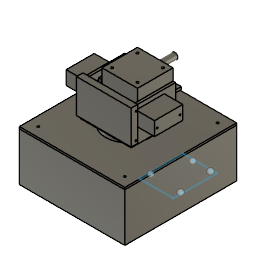
carro_armato_assieme_completo_modificabile_v3_batteria_integrata_canale_cavi (Autodesk Fusion 360 design; units mm, degrees)
part number: 2026-07-14-00-47-27-099
part number: 2026-07-14-00-47-27-347
part number: 2026-07-14-00-47-27-486
part number: 2026-07-14-00-47-29-459
part number: 2026-07-14-00-47-30-510
part number: 2026-07-14-00-47-30-620
part number: 2026-07-14-00-47-31-160
part number: 2026-07-14-00-47-33-248
part number: 2026-07-14-00-47-33-746
part number: 2026-07-14-00-47-35-683
part number: 2026-07-14-00-47-43-018
part number: 2026-07-14-00-47-43-807
part number: 2026-07-14-00-47-44-634
part number: 2026-07-14-00-47-46-224
part number: 2026-07-14-00-47-47-931
part number: 2026-07-14-00-47-54-379
part number: 2026-07-14-00-47-59-132
part number: 2026-07-14-00-48-06-266
part number: 2026-07-14-00-48-10-461
part number: 2026-07-14-00-48-14-735
Autodesk Fusion 360 part; units mm, degrees
(part 1 of 2)
sketch "Schizzo1" plane through (0, 0, 0) normal (0, 0, 1) x (1, 0, 0) in component "01_Piano_inferiore_colonnine_M3_supporto_batteria_integrato"
  line L0 (-80, -85) -> (80, -85)
  line L1 (80, -85) -> (80, 85)
  line L2 (80, 85) -> (-80, 85)
  line L3 (-80, 85) -> (-80, -85)
extrude "Estrusione_Piano_inferiore" add sketch "Schizzo1" along normal blind 3 makes body 1 in component "01_Piano_inferiore_colonnine_M3_supporto_batteria_integrato"
ref_plane "Piano di lavoro1" through (0, 0, 43) normal (0, 0, 1) x (1, 0, 0) in component "02_Piano_superiore"
sketch "Schizzo1 (2)" plane through (0, 0, 43) normal (0, 0, 1) x (1, 0, 0) in component "02_Piano_superiore"
  line L0 (-80, -85) -> (80, -85)
  line L1 (80, -85) -> (80, 85)
  line L2 (80, 85) -> (-80, 85)
  line L3 (-80, 85) -> (-80, -85)
extrude "Estrusione_Piano_superiore" add sketch "Schizzo1 (2)" along normal blind 3 separate body makes body 2 in component "02_Piano_superiore"
ref_plane "Piano di lavoro1" through (0, 0, 3) normal (0, 0, 1) x (1, 0, 0) in component "01_Piano_inferiore_colonnine_M3_supporto_batteria_integrato"
ref_plane "Piano di lavoro2" through (0, 0, 40.4) normal (0, 0, 1) x (1, 0, 0) in component "01_Piano_inferiore_colonnine_M3_supporto_batteria_integrato"
sketch "Schizzo2" plane through (0, 0, 0) normal (0, 0, 1) x (1, 0, 0) in component "01_Piano_inferiore_colonnine_M3_supporto_batteria_integrato"
  line L0 (-5, -77.5) -> (5, -77.5)
  line L1 (5, -77.5) -> (5, -72.5)
  line L2 (5, -72.5) -> (-5, -72.5)
  line L3 (-5, -72.5) -> (-5, -77.5)
extrude "Asola_fascetta_01" cut sketch "Schizzo2" along normal blind 3 bodies 1 in component "01_Piano_inferiore_colonnine_M3_supporto_batteria_integrato"
sketch "Schizzo3" plane through (0, 0, 0) normal (0, 0, 1) x (1, 0, 0) in component "01_Piano_inferiore_colonnine_M3_supporto_batteria_integrato"
  line L0 (-5, -62.5) -> (5, -62.5)
  line L1 (5, -62.5) -> (5, -57.5)
  line L2 (5, -57.5) -> (-5, -57.5)
  line L3 (-5, -57.5) -> (-5, -62.5)
extrude "Asola_fascetta_02" cut sketch "Schizzo3" along normal blind 3 bodies 1 in component "01_Piano_inferiore_colonnine_M3_supporto_batteria_integrato"
sketch "Schizzo4" plane through (0, 0, 0) normal (0, 0, 1) x (1, 0, 0) in component "01_Piano_inferiore_colonnine_M3_supporto_batteria_integrato"
  line L0 (-5, -12.5) -> (5, -12.5)
  line L1 (5, -12.5) -> (5, -7.5)
  line L2 (5, -7.5) -> (-5, -7.5)
  line L3 (-5, -7.5) -> (-5, -12.5)
extrude "Asola_fascetta_03" cut sketch "Schizzo4" along normal blind 3 bodies 1 in component "01_Piano_inferiore_colonnine_M3_supporto_batteria_integrato"
sketch "Schizzo5" plane through (0, 0, 0) normal (0, 0, 1) x (1, 0, 0) in component "01_Piano_inferiore_colonnine_M3_supporto_batteria_integrato"
  line L0 (-5, 2.5) -> (5, 2.5)
  line L1 (5, 2.5) -> (5, 7.5)
  line L2 (5, 7.5) -> (-5, 7.5)
  line L3 (-5, 7.5) -> (-5, 2.5)
extrude "Asola_fascetta_04" cut sketch "Schizzo5" along normal blind 3 bodies 1 in component "01_Piano_inferiore_colonnine_M3_supporto_batteria_integrato"
sketch "Schizzo2 (2)" plane through (0, 0, 43) normal (0, 0, 1) x (1, 0, 0) in component "02_Piano_superiore"
  circle A0 centre (-68, -73) radius 1.6
extrude "Foro_M3_superiore_01" cut sketch "Schizzo2 (2)" along normal blind 3 bodies 2 in component "02_Piano_superiore"
sketch "Schizzo6" plane through (0, 0, 3) normal (0, 0, 1) x (1, 0, 0) in component "01_Piano_inferiore_colonnine_M3_supporto_batteria_integrato"
  circle A0 centre (-68, -73) radius 5
extrude "Estrusione_Colonnina_M3_01" add sketch "Schizzo6" along normal blind 40 bodies 1 in component "01_Piano_inferiore_colonnine_M3_supporto_batteria_integrato"
sketch "Schizzo7" plane through (0, 0, 0) normal (0, 0, 1) x (1, 0, 0) in component "01_Piano_inferiore_colonnine_M3_supporto_batteria_integrato"
  circle A0 centre (-68, -73) radius 1.6
extrude "Foro_passante_M3_colonnina_01" cut sketch "Schizzo7" along normal blind 43 bodies 1 in component "01_Piano_inferiore_colonnine_M3_supporto_batteria_integrato"
sketch "Schizzo8" plane through (0, 0, 40.4) normal (0, 0, 1) x (1, 0, 0) in component "01_Piano_inferiore_colonnine_M3_supporto_batteria_integrato"
  line L0 (-65.1, -71.3257) -> (-68, -69.6514)
  line L1 (-68, -69.6514) -> (-70.9, -71.3257)
  line L2 (-70.9, -71.3257) -> (-70.9, -74.6743)
  line L3 (-70.9, -74.6743) -> (-68, -76.3486)
  line L4 (-68, -76.3486) -> (-65.1, -74.6743)
  line L5 (-65.1, -74.6743) -> (-65.1, -71.3257)
extrude "Sede_dado_M3_01" cut sketch "Schizzo8" along normal blind 2.6 bodies 1 in component "01_Piano_inferiore_colonnine_M3_supporto_batteria_integrato"
sketch "Schizzo3 (2)" plane through (0, 0, 43) normal (0, 0, 1) x (1, 0, 0) in component "02_Piano_superiore"
  circle A0 centre (68, -73) radius 1.6
extrude "Foro_M3_superiore_02" cut sketch "Schizzo3 (2)" along normal blind 3 bodies 2 in component "02_Piano_superiore"
sketch "Schizzo9" plane through (0, 0, 3) normal (0, 0, 1) x (1, 0, 0) in component "01_Piano_inferiore_colonnine_M3_supporto_batteria_integrato"
  circle A0 centre (68, -73) radius 5
extrude "Estrusione_Colonnina_M3_02" add sketch "Schizzo9" along normal blind 40 bodies 1 in component "01_Piano_inferiore_colonnine_M3_supporto_batteria_integrato"
sketch "Schizzo10" plane through (0, 0, 0) normal (0, 0, 1) x (1, 0, 0) in component "01_Piano_inferiore_colonnine_M3_supporto_batteria_integrato"
  circle A0 centre (68, -73) radius 1.6
extrude "Foro_passante_M3_colonnina_02" cut sketch "Schizzo10" along normal blind 43 bodies 1 in component "01_Piano_inferiore_colonnine_M3_supporto_batteria_integrato"
sketch "Schizzo11" plane through (0, 0, 40.4) normal (0, 0, 1) x (1, 0, 0) in component "01_Piano_inferiore_colonnine_M3_supporto_batteria_integrato"
  line L0 (70.9, -71.3257) -> (68, -69.6514)
  line L1 (68, -69.6514) -> (65.1, -71.3257)
  line L2 (65.1, -71.3257) -> (65.1, -74.6743)
  line L3 (65.1, -74.6743) -> (68, -76.3486)
  line L4 (68, -76.3486) -> (70.9, -74.6743)
  line L5 (70.9, -74.6743) -> (70.9, -71.3257)
extrude "Sede_dado_M3_02" cut sketch "Schizzo11" along normal blind 2.6 bodies 1 in component "01_Piano_inferiore_colonnine_M3_supporto_batteria_integrato"
sketch "Schizzo4 (2)" plane through (0, 0, 43) normal (0, 0, 1) x (1, 0, 0) in component "02_Piano_superiore"
  circle A0 centre (68, 73) radius 1.6
extrude "Foro_M3_superiore_03" cut sketch "Schizzo4 (2)" along normal blind 3 bodies 2 in component "02_Piano_superiore"
sketch "Schizzo12" plane through (0, 0, 3) normal (0, 0, 1) x (1, 0, 0) in component "01_Piano_inferiore_colonnine_M3_supporto_batteria_integrato"
  circle A0 centre (68, 73) radius 5
extrude "Estrusione_Colonnina_M3_03" add sketch "Schizzo12" along normal blind 40 bodies 1 in component "01_Piano_inferiore_colonnine_M3_supporto_batteria_integrato"
sketch "Schizzo13" plane through (0, 0, 0) normal (0, 0, 1) x (1, 0, 0) in component "01_Piano_inferiore_colonnine_M3_supporto_batteria_integrato"
  circle A0 centre (68, 73) radius 1.6
extrude "Foro_passante_M3_colonnina_03" cut sketch "Schizzo13" along normal blind 43 bodies 1 in component "01_Piano_inferiore_colonnine_M3_supporto_batteria_integrato"
sketch "Schizzo14" plane through (0, 0, 40.4) normal (0, 0, 1) x (1, 0, 0) in component "01_Piano_inferiore_colonnine_M3_supporto_batteria_integrato"
  line L0 (70.9, 74.6743) -> (68, 76.3486)
  line L1 (68, 76.3486) -> (65.1, 74.6743)
  line L2 (65.1, 74.6743) -> (65.1, 71.3257)
  line L3 (65.1, 71.3257) -> (68, 69.6514)
  line L4 (68, 69.6514) -> (70.9, 71.3257)
  line L5 (70.9, 71.3257) -> (70.9, 74.6743)
extrude "Sede_dado_M3_03" cut sketch "Schizzo14" along normal blind 2.6 bodies 1 in component "01_Piano_inferiore_colonnine_M3_supporto_batteria_integrato"
sketch "Schizzo5 (2)" plane through (0, 0, 43) normal (0, 0, 1) x (1, 0, 0) in component "02_Piano_superiore"
  circle A0 centre (-68, 73) radius 1.6
extrude "Foro_M3_superiore_04" cut sketch "Schizzo5 (2)" along normal blind 3 bodies 2 in component "02_Piano_superiore"
sketch "Schizzo15" plane through (0, 0, 3) normal (0, 0, 1) x (1, 0, 0) in component "01_Piano_inferiore_colonnine_M3_supporto_batteria_integrato"
  circle A0 centre (-68, 73) radius 5
extrude "Estrusione_Colonnina_M3_04" add sketch "Schizzo15" along normal blind 40 bodies 1 in component "01_Piano_inferiore_colonnine_M3_supporto_batteria_integrato"
sketch "Schizzo16" plane through (0, 0, 0) normal (0, 0, 1) x (1, 0, 0) in component "01_Piano_inferiore_colonnine_M3_supporto_batteria_integrato"
  circle A0 centre (-68, 73) radius 1.6
extrude "Foro_passante_M3_colonnina_04" cut sketch "Schizzo16" along normal blind 43 bodies 1 in component "01_Piano_inferiore_colonnine_M3_supporto_batteria_integrato"
sketch "Schizzo17" plane through (0, 0, 40.4) normal (0, 0, 1) x (1, 0, 0) in component "01_Piano_inferiore_colonnine_M3_supporto_batteria_integrato"
  line L0 (-65.1, 74.6743) -> (-68, 76.3486)
  line L1 (-68, 76.3486) -> (-70.9, 74.6743)
  line L2 (-70.9, 74.6743) -> (-70.9, 71.3257)
  line L3 (-70.9, 71.3257) -> (-68, 69.6514)
  line L4 (-68, 69.6514) -> (-65.1, 71.3257)
  line L5 (-65.1, 71.3257) -> (-65.1, 74.6743)
extrude "Sede_dado_M3_04" cut sketch "Schizzo17" along normal blind 2.6 bodies 1 in component "01_Piano_inferiore_colonnine_M3_supporto_batteria_integrato"
sketch "Schizzo6 (2)" plane through (0, 0, 43) normal (0, 0, 1) x (1, 0, 0) in component "02_Piano_superiore"
  line L0 (20.83, 33.21) -> (45.83, 33.21)
  line L1 (45.83, 33.21) -> (45.83, 58.21)
  line L2 (45.83, 58.21) -> (20.83, 58.21)
  line L3 (20.83, 58.21) -> (20.83, 33.21)
extrude "Apertura_Arduino_25x25_D2_D7_S1_S8" cut sketch "Schizzo6 (2)" along normal blind 3 bodies 2 in component "02_Piano_superiore"
sketch "Schizzo7 (2)" plane through (0, 0, 43) normal (0, 0, 1) x (1, 0, 0) in component "02_Piano_superiore"
  line L0 (-69, -45) -> (-36, -45)
  line L1 (-36, -45) -> (-36, 15)
  line L2 (-36, 15) -> (-69, 15)
  line L3 (-69, 15) -> (-69, -45)
extrude "Apertura_pacco_batteria_PCB_cannone_60x33" cut sketch "Schizzo7 (2)" along normal blind 3 bodies 2 in component "02_Piano_superiore"
sketch "Schizzo8 (2)" plane through (0, 0, 43) normal (0, 0, 1) x (1, 0, 0) in component "02_Piano_superiore"
  circle A0 centre (0, -79.5) radius 1.35
extrude "Foro_M2_5_guscio_inferiore_01_south" cut sketch "Schizzo8 (2)" along normal blind 3 bodies 2 in component "02_Piano_superiore"
sketch "Schizzo9 (2)" plane through (0, 0, 43) normal (0, 0, 1) x (1, 0, 0) in component "02_Piano_superiore"
  circle A0 centre (0, 79.5) radius 1.35
extrude "Foro_M2_5_guscio_inferiore_02_north" cut sketch "Schizzo9 (2)" along normal blind 3 bodies 2 in component "02_Piano_superiore"
sketch "Schizzo10 (2)" plane through (0, 0, 43) normal (0, 0, 1) x (1, 0, 0) in component "02_Piano_superiore"
  circle A0 centre (74.5, 45) radius 1.35
extrude "Foro_M2_5_guscio_inferiore_03_east" cut sketch "Schizzo10 (2)" along normal blind 3 bodies 2 in component "02_Piano_superiore"
sketch "Schizzo11 (2)" plane through (0, 0, 43) normal (0, 0, 1) x (1, 0, 0) in component "02_Piano_superiore"
  circle A0 centre (-74.5, 45) radius 1.35
extrude "Foro_M2_5_guscio_inferiore_04_west" cut sketch "Schizzo11 (2)" along normal blind 3 bodies 2 in component "02_Piano_superiore"
ref_plane "Piano di lavoro3" through (0, 0, 3) normal (0, 0, 1) x (1, 0, 0) in component "01_Piano_inferiore_colonnine_M3_supporto_batteria_integrato"
sketch "Schizzo18" plane through (0, 0, 3) normal (0, 0, 1) x (1, 0, 0) in component "01_Piano_inferiore_colonnine_M3_supporto_batteria_integrato"
  line L0 (-75, -65) -> (-72.5, -65)
  line L1 (-72.5, -65) -> (-72.5, 35)
  line L2 (-72.5, 35) -> (-75, 35)
  line L3 (-75, 35) -> (-75, -65)
extrude "Estrusione_Parete_lunga_Ovest" add sketch "Schizzo18" along normal blind 17 bodies 1 in component "01_Piano_inferiore_colonnine_M3_supporto_batteria_integrato"
sketch "Schizzo19" plane through (0, 0, 3) normal (0, 0, 1) x (1, 0, 0) in component "01_Piano_inferiore_colonnine_M3_supporto_batteria_integrato"
  line L0 (-32.5, -65) -> (-30, -65)
  line L1 (-30, -65) -> (-30, 35)
  line L2 (-30, 35) -> (-32.5, 35)
  line L3 (-32.5, 35) -> (-32.5, -65)
extrude "Estrusione_Parete_lunga_Est" add sketch "Schizzo19" along normal blind 17 bodies 1 in component "01_Piano_inferiore_colonnine_M3_supporto_batteria_integrato"
sketch "Schizzo20" plane through (0, 0, 3) normal (0, 0, 1) x (1, 0, 0) in component "01_Piano_inferiore_colonnine_M3_supporto_batteria_integrato"
  line L0 (-75, -65) -> (-30, -65)
  line L1 (-30, -65) -> (-30, -60)
  line L2 (-30, -60) -> (-75, -60)
  line L3 (-75, -60) -> (-75, -65)
extrude "Estrusione_Parete_corta_chiusa" add sketch "Schizzo20" along normal blind 17 bodies 1 in component "01_Piano_inferiore_colonnine_M3_supporto_batteria_integrato"
sketch "Schizzo21" plane through (0, 0, 3) normal (0, 0, 1) x (1, 0, 0) in component "01_Piano_inferiore_colonnine_M3_supporto_batteria_integrato"
  line L0 (-32.6, -60) -> (-29.9, -60)
  line L1 (-29.9, -60) -> (-29.9, -50)
  line L2 (-29.9, -50) -> (-32.6, -50)
  line L3 (-32.6, -50) -> (-32.6, -60)
extrude "Apertura_cavi_parete_lunga_Est" cut sketch "Schizzo21" along normal blind 17 bodies 1 in component "01_Piano_inferiore_colonnine_M3_supporto_batteria_integrato"
sketch "Schizzo1 (3)" plane through (0, 0, 0) normal (0, 0, 1) x (1, 0, 0) in component "03_Guscio_laterale_continuo_carro"
  line L0 (-83, -88) -> (-80.5, -88)
  line L1 (-80.5, -88) -> (-80.5, 88)
  line L2 (-80.5, 88) -> (-83, 88)
  line L3 (-83, 88) -> (-83, -88)
extrude "Estrusione_Parete_guscio_Ovest" add sketch "Schizzo1 (3)" along normal blind 76 separate body makes body 3 in component "03_Guscio_laterale_continuo_carro"
sketch "Schizzo2 (3)" plane through (0, 0, 0) normal (0, 0, 1) x (1, 0, 0) in component "03_Guscio_laterale_continuo_carro"
  line L0 (-83, -88) -> (83, -88)
  line L1 (83, -88) -> (83, -85.5)
  line L2 (83, -85.5) -> (-83, -85.5)
  line L3 (-83, -85.5) -> (-83, -88)
extrude "Estrusione_Parete_guscio_Sud" add sketch "Schizzo2 (3)" along normal blind 76 bodies 3 in component "03_Guscio_laterale_continuo_carro"
sketch "Schizzo3 (3)" plane through (0, 0, 0) normal (0, 0, 1) x (1, 0, 0) in component "03_Guscio_laterale_continuo_carro"
  line L0 (80.5, -88) -> (83, -88)
  line L1 (83, -88) -> (83, 88)
  line L2 (83, 88) -> (80.5, 88)
  line L3 (80.5, 88) -> (80.5, -88)
extrude "Estrusione_Parete_guscio_Est" add sketch "Schizzo3 (3)" along normal blind 76 bodies 3 in component "03_Guscio_laterale_continuo_carro"
sketch "Schizzo4 (3)" plane through (0, 0, 0) normal (0, 0, 1) x (1, 0, 0) in component "03_Guscio_laterale_continuo_carro"
  line L0 (-83, 85.5) -> (83, 85.5)
  line L1 (83, 85.5) -> (83, 88)
  line L2 (83, 88) -> (-83, 88)
  line L3 (-83, 88) -> (-83, 85.5)
extrude "Estrusione_Parete_guscio_Nord" add sketch "Schizzo4 (3)" along normal blind 76 bodies 3 in component "03_Guscio_laterale_continuo_carro"
ref_plane "Piano di lavoro1" through (0, 0, 38) normal (0, 0, 1) x (1, 0, 0) in component "03_Guscio_laterale_continuo_carro"
sketch "Schizzo5 (3)" plane through (0, 0, 38) normal (0, 0, 1) x (1, 0, 0) in component "03_Guscio_laterale_continuo_carro"
  line L0 (-7, -86) -> (7, -86)
  line L1 (7, -86) -> (7, -73)
  line L2 (7, -73) -> (-7, -73)
  line L3 (-7, -73) -> (-7, -86)
extrude "Estrusione_Linguetta_M2_5_01_south" add sketch "Schizzo5 (3)" along normal blind 5 bodies 3 in component "03_Guscio_laterale_continuo_carro"
sketch "Schizzo6 (3)" plane through (0, 0, 38) normal (0, 0, 1) x (1, 0, 0) in component "03_Guscio_laterale_continuo_carro"
  circle A0 centre (0, -79.5) radius 1.1
extrude "Preforo_M2_5_guscio_01_south" cut sketch "Schizzo6 (3)" along normal blind 5 bodies 3 in component "03_Guscio_laterale_continuo_carro"
sketch "Schizzo7 (3)" plane through (0, 0, 38) normal (0, 0, 1) x (1, 0, 0) in component "03_Guscio_laterale_continuo_carro"
  line L0 (-7, 73) -> (7, 73)
  line L1 (7, 73) -> (7, 86)
  line L2 (7, 86) -> (-7, 86)
  line L3 (-7, 86) -> (-7, 73)
extrude "Estrusione_Linguetta_M2_5_02_north" add sketch "Schizzo7 (3)" along normal blind 5 bodies 3 in component "03_Guscio_laterale_continuo_carro"
sketch "Schizzo8 (3)" plane through (0, 0, 38) normal (0, 0, 1) x (1, 0, 0) in component "03_Guscio_laterale_continuo_carro"
  circle A0 centre (0, 79.5) radius 1.1
extrude "Preforo_M2_5_guscio_02_north" cut sketch "Schizzo8 (3)" along normal blind 5 bodies 3 in component "03_Guscio_laterale_continuo_carro"
sketch "Schizzo9 (3)" plane through (0, 0, 38) normal (0, 0, 1) x (1, 0, 0) in component "03_Guscio_laterale_continuo_carro"
  line L0 (68, 38) -> (81, 38)
  line L1 (81, 38) -> (81, 52)
  line L2 (81, 52) -> (68, 52)
  line L3 (68, 52) -> (68, 38)
extrude "Estrusione_Linguetta_M2_5_03_east" add sketch "Schizzo9 (3)" along normal blind 5 bodies 3 in component "03_Guscio_laterale_continuo_carro"
sketch "Schizzo10 (3)" plane through (0, 0, 38) normal (0, 0, 1) x (1, 0, 0) in component "03_Guscio_laterale_continuo_carro"
  circle A0 centre (74.5, 45) radius 1.1
extrude "Preforo_M2_5_guscio_03_east" cut sketch "Schizzo10 (3)" along normal blind 5 bodies 3 in component "03_Guscio_laterale_continuo_carro"
sketch "Schizzo11 (3)" plane through (0, 0, 38) normal (0, 0, 1) x (1, 0, 0) in component "03_Guscio_laterale_continuo_carro"
  line L0 (-81, 38) -> (-68, 38)
  line L1 (-68, 38) -> (-68, 52)
  line L2 (-68, 52) -> (-81, 52)
  line L3 (-81, 52) -> (-81, 38)
extrude "Estrusione_Linguetta_M2_5_04_west" add sketch "Schizzo11 (3)" along normal blind 5 bodies 3 in component "03_Guscio_laterale_continuo_carro"
sketch "Schizzo12 (2)" plane through (0, 0, 38) normal (0, 0, 1) x (1, 0, 0) in component "03_Guscio_laterale_continuo_carro"
  circle A0 centre (-74.5, 45) radius 1.1
extrude "Preforo_M2_5_guscio_04_west" cut sketch "Schizzo12 (2)" along normal blind 5 bodies 3 in component "03_Guscio_laterale_continuo_carro"
sketch "Schizzo1 (4)" plane through (0, 0, 0) normal (0, 0, 1) x (1, 0, 0) in component "05_Arduino_UNO_R4_WiFi_RIFERIMENTO_XY_quota_Z_da_definire"
  line L0 (-26.67, -34.29) -> (26.67, -34.29)
  line L1 (26.67, -34.29) -> (26.67, 34.29)
  line L2 (26.67, 34.29) -> (-26.67, 34.29)
  line L3 (-26.67, 34.29) -> (-26.67, -34.29)
  circle A0 centre (24.13, -20.32) radius 1.6
  circle A1 centre (-24.13, -19.05) radius 1.6
  circle A2 centre (19.05, 31.75) radius 1.6
  circle A3 centre (-8.89, 31.75) radius 1.6
ref_plane "Piano di lavoro1" through (0, 0, 30) normal (0, 0, 1) x (1, 0, 0) in component "01_Tetto_elettronica_removibile"
sketch "Schizzo1 (5)" plane through (0, 0, 30) normal (0, 0, 1) x (1, 0, 0) in component "01_Tetto_elettronica_removibile"
  line L0 (-83, -88) -> (83, -88)
  line L1 (83, -88) -> (83, 88)
  line L2 (83, 88) -> (-83, 88)
  line L3 (-83, 88) -> (-83, -88)
extrude "Estrusione_Tetto_coperchio" add sketch "Schizzo1 (5)" along normal blind 3 separate body makes body 4 in component "01_Tetto_elettronica_removibile"
sketch "Schizzo2 (4)" plane through (0, 0, 0) normal (0, 0, 1) x (1, 0, 0) in component "01_Tetto_elettronica_removibile"
  circle A0 centre (-68, -73) radius 5
extrude "Estrusione_Boss_verticale_M3_coperchio_01" add sketch "Schizzo2 (4)" along normal blind 33 bodies 4 in component "01_Tetto_elettronica_removibile"
sketch "Schizzo3 (4)" plane through (0, 0, 0) normal (0, 0, 1) x (1, 0, 0) in component "01_Tetto_elettronica_removibile"
  circle A0 centre (-68, -73) radius 1.6
extrude "Foro_M3_accessibile_dal_tetto_01" cut sketch "Schizzo3 (4)" along normal blind 33 bodies 4 in component "01_Tetto_elettronica_removibile"
sketch "Schizzo4 (4)" plane through (0, 0, 0) normal (0, 0, 1) x (1, 0, 0) in component "01_Tetto_elettronica_removibile"
  circle A0 centre (68, -73) radius 5
extrude "Estrusione_Boss_verticale_M3_coperchio_02" add sketch "Schizzo4 (4)" along normal blind 33 bodies 4 in component "01_Tetto_elettronica_removibile"
sketch "Schizzo5 (4)" plane through (0, 0, 0) normal (0, 0, 1) x (1, 0, 0) in component "01_Tetto_elettronica_removibile"
  circle A0 centre (68, -73) radius 1.6
extrude "Foro_M3_accessibile_dal_tetto_02" cut sketch "Schizzo5 (4)" along normal blind 33 bodies 4 in component "01_Tetto_elettronica_removibile"
sketch "Schizzo6 (4)" plane through (0, 0, 0) normal (0, 0, 1) x (1, 0, 0) in component "01_Tetto_elettronica_removibile"
  circle A0 centre (-68, 73) radius 5
extrude "Estrusione_Boss_verticale_M3_coperchio_03" add sketch "Schizzo6 (4)" along normal blind 33 bodies 4 in component "01_Tetto_elettronica_removibile"
sketch "Schizzo7 (4)" plane through (0, 0, 0) normal (0, 0, 1) x (1, 0, 0) in component "01_Tetto_elettronica_removibile"
  circle A0 centre (-68, 73) radius 1.6
extrude "Foro_M3_accessibile_dal_tetto_03" cut sketch "Schizzo7 (4)" along normal blind 33 bodies 4 in component "01_Tetto_elettronica_removibile"
sketch "Schizzo8 (4)" plane through (0, 0, 0) normal (0, 0, 1) x (1, 0, 0) in component "01_Tetto_elettronica_removibile"
  circle A0 centre (68, 73) radius 5
extrude "Estrusione_Boss_verticale_M3_coperchio_04" add sketch "Schizzo8 (4)" along normal blind 33 bodies 4 in component "01_Tetto_elettronica_removibile"
sketch "Schizzo9 (4)" plane through (0, 0, 0) normal (0, 0, 1) x (1, 0, 0) in component "01_Tetto_elettronica_removibile"
  circle A0 centre (68, 73) radius 1.6
extrude "Foro_M3_accessibile_dal_tetto_04" cut sketch "Schizzo9 (4)" along normal blind 33 bodies 4 in component "01_Tetto_elettronica_removibile"
ref_plane "Piano di lavoro2" through (0, 0, 30) normal (0, 0, 1) x (1, 0, 0) in component "01_Tetto_elettronica_removibile"
sketch "Schizzo10 (4)" plane through (0, 0, 30) normal (0, 0, 1) x (1, 0, 0) in component "01_Tetto_elettronica_removibile"
  circle A0 centre (0, 0) radius 4
extrude "Passaggio_albero_stepper" cut sketch "Schizzo10 (4)" along normal blind 3 bodies 4 in component "01_Tetto_elettronica_removibile"
sketch "Schizzo11 (4)" plane through (0, 0, 30) normal (0, 0, 1) x (1, 0, 0) in component "01_Tetto_elettronica_removibile"
  circle A0 centre (-17.5, 0) radius 2.1
extrude "Foro_stepper_Ovest" cut sketch "Schizzo11 (4)" along normal blind 3 bodies 4 in component "01_Tetto_elettronica_removibile"
sketch "Schizzo12 (3)" plane through (0, 0, 30) normal (0, 0, 1) x (1, 0, 0) in component "01_Tetto_elettronica_removibile"
  circle A0 centre (17.5, 0) radius 2.1
extrude "Foro_stepper_Est" cut sketch "Schizzo12 (3)" along normal blind 3 bodies 4 in component "01_Tetto_elettronica_removibile"
ref_plane "Piano di lavoro3" through (0, 0, 22.8) normal (0, 0, 1) x (1, 0, 0) in component "01_Tetto_elettronica_removibile"
sketch "Schizzo13 (2)" plane through (0, 0, 22.8) normal (0, 0, 1) x (1, 0, 0) in component "01_Tetto_elettronica_removibile"
  circle A0 centre (0, 0) radius 24
  circle A1 centre (0, 0) radius 22.5
extrude "Estrusione_Parete_interna_liscia_canale_cavi" add sketch "Schizzo13 (2)" along normal blind 7.4 bodies 4 in component "01_Tetto_elettronica_removibile"
sketch "Schizzo14 (2)" plane through (0, 0, 22.8) normal (0, 0, 1) x (1, 0, 0) in component "01_Tetto_elettronica_removibile"
  circle A0 centre (0, 0) radius 33.5
  circle A1 centre (0, 0) radius 32
extrude "Estrusione_Parete_esterna_liscia_canale_cavi" add sketch "Schizzo14 (2)" along normal blind 7.4 bodies 4 in component "01_Tetto_elettronica_removibile"
ref_plane "Piano di lavoro4" through (0, 0, 20) normal (0, 0, 1) x (1, 0, 0) in component "01_Tetto_elettronica_removibile"
sketch "Schizzo15 (2)" plane through (0, 0, 20) normal (0, 0, 1) x (1, 0, 0) in component "01_Tetto_elettronica_removibile"
  circle A0 centre (0, 0) radius 40
  circle A1 centre (0, 0) radius 19
extrude "Estrusione_Fondo_anulare_continuo_canale_cavi" add sketch "Schizzo15 (2)" along normal blind 3 bodies 4 in component "01_Tetto_elettronica_removibile"
sketch "Schizzo16 (2)" plane through (0, 0, 20) normal (0, 0, 1) x (1, 0, 0) in component "01_Tetto_elettronica_removibile"
  line L0 (19.0919, 14.8492) -> (24.7487, 20.5061)
  line L1 (24.7487, 20.5061) -> (20.5061, 24.7487)
  line L2 (20.5061, 24.7487) -> (14.8492, 19.0919)
  line L3 (14.8492, 19.0919) -> (19.0919, 14.8492)
extrude "Uscita_fissa_8x6_canale_cavi_verso_vano_elettronica" cut sketch "Schizzo16 (2)" along normal blind 3 bodies 4 in component "01_Tetto_elettronica_removibile"
sketch "Schizzo17 (2)" plane through (0, 0, 30) normal (0, 0, 1) x (1, 0, 0) in component "01_Tetto_elettronica_removibile"
  circle A0 centre (0, 0) radius 32
  circle A1 centre (0, 0) radius 24
extrude "Guida_anulare_cavi_azimut_meno180_piu180" cut sketch "Schizzo17 (2)" along normal blind 3 bodies 4 in component "01_Tetto_elettronica_removibile"
ref_plane "Piano di lavoro1" through (0, 0, 10) normal (0, 0, 1) x (1, 0, 0) in component "02_Stepper_28BYJ48_riferimento"
sketch "Schizzo1 (6)" plane through (0, 0, 10) normal (0, 0, 1) x (1, 0, 0) in component "02_Stepper_28BYJ48_riferimento"
  circle A0 centre (0, 0) radius 14
extrude "Estrusione_Corpo_stepper" add sketch "Schizzo1 (6)" along normal blind 20 separate body makes body 5 in component "02_Stepper_28BYJ48_riferimento"
ref_plane "Piano di lavoro2" through (0, 0, 27) normal (0, 0, 1) x (1, 0, 0) in component "02_Stepper_28BYJ48_riferimento"
sketch "Schizzo2 (5)" plane through (0, 0, 27) normal (0, 0, 1) x (1, 0, 0) in component "02_Stepper_28BYJ48_riferimento"
  line L0 (-20.75, -4) -> (20.75, -4)
  line L1 (20.75, -4) -> (20.75, 4)
  line L2 (20.75, 4) -> (-20.75, 4)
  line L3 (-20.75, 4) -> (-20.75, -4)
extrude "Estrusione_Alette_fissaggio_stepper" add sketch "Schizzo2 (5)" along normal blind 3 bodies 5 in component "02_Stepper_28BYJ48_riferimento"
ref_plane "Piano di lavoro3" through (0, 0, 30) normal (0, 0, 1) x (1, 0, 0) in component "02_Stepper_28BYJ48_riferimento"
sketch "Schizzo3 (5)" plane through (0, 0, 30) normal (0, 0, 1) x (1, 0, 0) in component "02_Stepper_28BYJ48_riferimento"
  circle A0 centre (0, 0) radius 2.5
extrude "Estrusione_Albero_stepper" add sketch "Schizzo3 (5)" along normal blind 9 bodies 5 in component "02_Stepper_28BYJ48_riferimento"
ref_plane "Piano di lavoro1" through (0, 0, 33) normal (0, 0, 1) x (1, 0, 0) in component "03_Adattatore_rotante_stepper"
sketch "Schizzo1 (7)" plane through (0, 0, 33) normal (0, 0, 1) x (1, 0, 0) in component "03_Adattatore_rotante_stepper"
  circle A0 centre (0, 0) radius 35
extrude "Estrusione_Piastra_adattatore_rotante" add sketch "Schizzo1 (7)" along normal blind 6 separate body makes body 6 in component "03_Adattatore_rotante_stepper"
sketch "Schizzo2 (6)" plane through (0, 0, 33) normal (0, 0, 1) x (1, 0, 0) in component "03_Adattatore_rotante_stepper"
  circle A0 centre (0, 0) radius 2.65
extrude "Sede_albero_stepper" cut sketch "Schizzo2 (6)" along normal blind 6 bodies 5 in component "02_Stepper_28BYJ48_riferimento"
extrude "Estrusione2" cut sketch "Schizzo2 (6)" along normal blind 6 bodies 6 in component "03_Adattatore_rotante_stepper"
ref_plane "Piano di lavoro2" through (0, 0, 36.4) normal (0, 0, 1) x (1, 0, 0) in component "03_Adattatore_rotante_stepper"
sketch "Schizzo3 (6)" plane through (0, 0, 33) normal (0, 0, 1) x (1, 0, 0) in component "03_Adattatore_rotante_stepper"
  circle A0 centre (-25, 0) radius 1.6
extrude "Foro_M3_adattatore_01" cut sketch "Schizzo3 (6)" along normal blind 6 bodies 6 in component "03_Adattatore_rotante_stepper"
sketch "Schizzo4 (5)" plane through (0, 0, 36.4) normal (0, 0, 1) x (1, 0, 0) in component "03_Adattatore_rotante_stepper"
  line L0 (-22.1, 1.6743) -> (-25, 3.3486)
  line L1 (-25, 3.3486) -> (-27.9, 1.6743)
  line L2 (-27.9, 1.6743) -> (-27.9, -1.6743)
  line L3 (-27.9, -1.6743) -> (-25, -3.3486)
  line L4 (-25, -3.3486) -> (-22.1, -1.6743)
  line L5 (-22.1, -1.6743) -> (-22.1, 1.6743)
extrude "Sede_dado_M3_adattatore_01" cut sketch "Schizzo4 (5)" along normal blind 2.6 bodies 6 in component "03_Adattatore_rotante_stepper"
sketch "Schizzo5 (5)" plane through (0, 0, 33) normal (0, 0, 1) x (1, 0, 0) in component "03_Adattatore_rotante_stepper"
  circle A0 centre (25, 0) radius 1.6
extrude "Foro_M3_adattatore_02" cut sketch "Schizzo5 (5)" along normal blind 6 bodies 6 in component "03_Adattatore_rotante_stepper"
sketch "Schizzo6 (5)" plane through (0, 0, 36.4) normal (0, 0, 1) x (1, 0, 0) in component "03_Adattatore_rotante_stepper"
  line L0 (27.9, 1.6743) -> (25, 3.3486)
  line L1 (25, 3.3486) -> (22.1, 1.6743)
  line L2 (22.1, 1.6743) -> (22.1, -1.6743)
  line L3 (22.1, -1.6743) -> (25, -3.3486)
  line L4 (25, -3.3486) -> (27.9, -1.6743)
  line L5 (27.9, -1.6743) -> (27.9, 1.6743)
extrude "Sede_dado_M3_adattatore_02" cut sketch "Schizzo6 (5)" along normal blind 2.6 bodies 6 in component "03_Adattatore_rotante_stepper"
sketch "Schizzo7 (5)" plane through (0, 0, 33) normal (0, 0, 1) x (1, 0, 0) in component "03_Adattatore_rotante_stepper"
  circle A0 centre (0, -25) radius 1.6
extrude "Foro_M3_adattatore_03" cut sketch "Schizzo7 (5)" along normal blind 6 bodies 6 in component "03_Adattatore_rotante_stepper"
sketch "Schizzo8 (5)" plane through (0, 0, 36.4) normal (0, 0, 1) x (1, 0, 0) in component "03_Adattatore_rotante_stepper"
  line L0 (2.9, -23.3257) -> (0, -21.6514)
  line L1 (0, -21.6514) -> (-2.9, -23.3257)
  line L2 (-2.9, -23.3257) -> (-2.9, -26.6743)
  line L3 (-2.9, -26.6743) -> (0, -28.3486)
  line L4 (0, -28.3486) -> (2.9, -26.6743)
  line L5 (2.9, -26.6743) -> (2.9, -23.3257)
extrude "Sede_dado_M3_adattatore_03" cut sketch "Schizzo8 (5)" along normal blind 2.6 bodies 6 in component "03_Adattatore_rotante_stepper"
sketch "Schizzo9 (5)" plane through (0, 0, 33) normal (0, 0, 1) x (1, 0, 0) in component "03_Adattatore_rotante_stepper"
  circle A0 centre (0, 25) radius 1.6
extrude "Foro_M3_adattatore_04" cut sketch "Schizzo9 (5)" along normal blind 6 bodies 6 in component "03_Adattatore_rotante_stepper"
sketch "Schizzo10 (5)" plane through (0, 0, 36.4) normal (0, 0, 1) x (1, 0, 0) in component "03_Adattatore_rotante_stepper"
  line L0 (2.9, 26.6743) -> (0, 28.3486)
  line L1 (0, 28.3486) -> (-2.9, 26.6743)
  line L2 (-2.9, 26.6743) -> (-2.9, 23.3257)
  line L3 (-2.9, 23.3257) -> (0, 21.6514)
  line L4 (0, 21.6514) -> (2.9, 23.3257)
  line L5 (2.9, 23.3257) -> (2.9, 26.6743)
extrude "Sede_dado_M3_adattatore_04" cut sketch "Schizzo10 (5)" along normal blind 2.6 bodies 6 in component "03_Adattatore_rotante_stepper"
sketch "Schizzo11 (5)" plane through (0, 0, 33) normal (0, 0, 1) x (1, 0, 0) in component "03_Adattatore_rotante_stepper"
  line L0 (19.0919, 14.8492) -> (24.7487, 20.5061)
  line L1 (24.7487, 20.5061) -> (20.5061, 24.7487)
  line L2 (20.5061, 24.7487) -> (14.8492, 19.0919)
  line L3 (14.8492, 19.0919) -> (19.0919, 14.8492)
extrude "Passaggio_8x6_comune_servi_cannone_adattatore" cut sketch "Schizzo11 (5)" along normal blind 6 bodies 6 in component "03_Adattatore_rotante_stepper"
ref_plane "Piano di lavoro1" through (0, 0, 39) normal (0, 0, 1) x (1, 0, 0) in component "04_Torretta_parte_fissa_azimut"
sketch "Schizzo1 (8)" plane through (0, 0, 39) normal (0, 0, 1) x (1, 0, 0) in component "04_Torretta_parte_fissa_azimut"
  line L0 (-40, -35) -> (40, -35)
  line L1 (40, -35) -> (40, 35)
  line L2 (40, 35) -> (-40, 35)
  line L3 (-40, 35) -> (-40, -35)
extrude "Estrusione_Base_parte_fissa" add sketch "Schizzo1 (8)" along normal blind 4 separate body makes body 7 in component "04_Torretta_parte_fissa_azimut"
sketch "Schizzo2 (7)" plane through (0, 0, 39) normal (0, 0, 1) x (1, 0, 0) in component "04_Torretta_parte_fissa_azimut"
  circle A0 centre (-25, 0) radius 1.6
extrude "Foro_M3_base_fissa_01" cut sketch "Schizzo2 (7)" along normal blind 4 bodies 7 in component "04_Torretta_parte_fissa_azimut"
sketch "Schizzo3 (7)" plane through (0, 0, 39) normal (0, 0, 1) x (1, 0, 0) in component "04_Torretta_parte_fissa_azimut"
  circle A0 centre (25, 0) radius 1.6
extrude "Foro_M3_base_fissa_02" cut sketch "Schizzo3 (7)" along normal blind 4 bodies 7 in component "04_Torretta_parte_fissa_azimut"
sketch "Schizzo4 (6)" plane through (0, 0, 39) normal (0, 0, 1) x (1, 0, 0) in component "04_Torretta_parte_fissa_azimut"
  circle A0 centre (0, -25) radius 1.6
extrude "Foro_M3_base_fissa_03" cut sketch "Schizzo4 (6)" along normal blind 4 bodies 7 in component "04_Torretta_parte_fissa_azimut"
sketch "Schizzo5 (6)" plane through (0, 0, 39) normal (0, 0, 1) x (1, 0, 0) in component "04_Torretta_parte_fissa_azimut"
  circle A0 centre (0, 25) radius 1.6
extrude "Foro_M3_base_fissa_04" cut sketch "Schizzo5 (6)" along normal blind 4 bodies 7 in component "04_Torretta_parte_fissa_azimut"
sketch "Schizzo6 (6)" plane through (0, 0, 39) normal (0, 0, 1) x (1, 0, 0) in component "04_Torretta_parte_fissa_azimut"
  line L0 (19.0919, 14.8492) -> (24.7487, 20.5061)
  line L1 (24.7487, 20.5061) -> (20.5061, 24.7487)
  line L2 (20.5061, 24.7487) -> (14.8492, 19.0919)
  line L3 (14.8492, 19.0919) -> (19.0919, 14.8492)
extrude "Passaggio_8x6_comune_servi_cannone_base_fissa" cut sketch "Schizzo6 (6)" along normal blind 4 bodies 7 in component "04_Torretta_parte_fissa_azimut"
ref_plane "Piano di lavoro2" through (-40, 0, 0) normal (1, 0, 0) x (0, 1, 0) in component "04_Torretta_parte_fissa_azimut"
sketch "Schizzo7 (6)" plane through (-40, 0, 0) normal (1, 0, 0) x (0, 0, -1) in component "04_Torretta_parte_fissa_azimut"
  line L0 (-43, -35) -> (-93, -35)
  line L1 (-93, -35) -> (-93, 35)
  line L2 (-93, 35) -> (-43, 35)
  line L3 (-43, 35) -> (-43, -35)
extrude "Estrusione_Parete_fissa_Sinistra" add sketch "Schizzo7 (6)" along normal blind 4 bodies 7 in component "04_Torretta_parte_fissa_azimut"
ref_plane "Piano di lavoro3" through (-40, 0, 0) normal (1, 0, 0) x (0, 1, 0) in component "04_Torretta_parte_fissa_azimut"
sketch "Schizzo8 (6)" plane through (-40, 0, 0) normal (1, 0, 0) x (0, 0, -1) in component "04_Torretta_parte_fissa_azimut"
  line L0 (-68.4, -17.5) -> (-81.6, -17.5)
  line L1 (-81.6, -17.5) -> (-81.6, 6.2)
  line L2 (-81.6, 6.2) -> (-68.4, 6.2)
  line L3 (-68.4, 6.2) -> (-68.4, -17.5)
extrude "Finestra_inserimento_SG90_Sinistra" cut sketch "Schizzo8 (6)" along normal blind 4 bodies 7 in component "04_Torretta_parte_fissa_azimut"
ref_plane "Piano di lavoro4" through (-40, 0, 0) normal (1, 0, 0) x (0, 1, 0) in component "04_Torretta_parte_fissa_azimut"
sketch "Schizzo9 (6)" plane through (-40, 0, 0) normal (1, 0, 0) x (0, 0, -1) in component "04_Torretta_parte_fissa_azimut"
  line L0 (-63.9, -8.15) -> (-68.4, -8.15)
  line L1 (-68.4, -8.15) -> (-68.4, -3.15)
  line L2 (-68.4, -3.15) -> (-63.9, -3.15)
  line L3 (-63.9, -3.15) -> (-63.9, -8.15)
extrude "Diramazione_cavo_5x4_5_SG90_Sinistra" cut sketch "Schizzo9 (6)" along normal blind 4 bodies 7 in component "04_Torretta_parte_fissa_azimut"
ref_plane "Piano di lavoro5" through (36, 0, 0) normal (1, 0, 0) x (0, 1, 0) in component "04_Torretta_parte_fissa_azimut"
sketch "Schizzo10 (6)" plane through (36, 0, 0) normal (1, 0, 0) x (0, 0, -1) in component "04_Torretta_parte_fissa_azimut"
  line L0 (-43, -35) -> (-93, -35)
  line L1 (-93, -35) -> (-93, 35)
  line L2 (-93, 35) -> (-43, 35)
  line L3 (-43, 35) -> (-43, -35)
extrude "Estrusione_Parete_fissa_Destra" add sketch "Schizzo10 (6)" along normal blind 4 bodies 7 in component "04_Torretta_parte_fissa_azimut"
ref_plane "Piano di lavoro6" through (36, 0, 0) normal (1, 0, 0) x (0, 1, 0) in component "04_Torretta_parte_fissa_azimut"
sketch "Schizzo11 (6)" plane through (36, 0, 0) normal (1, 0, 0) x (0, 0, -1) in component "04_Torretta_parte_fissa_azimut"
  line L0 (-68.4, -17.5) -> (-81.6, -17.5)
  line L1 (-81.6, -17.5) -> (-81.6, 6.2)
  line L2 (-81.6, 6.2) -> (-68.4, 6.2)
  line L3 (-68.4, 6.2) -> (-68.4, -17.5)
extrude "Finestra_inserimento_SG90_Destra" cut sketch "Schizzo11 (6)" along normal blind 4 bodies 7 in component "04_Torretta_parte_fissa_azimut"
ref_plane "Piano di lavoro7" through (36, 0, 0) normal (1, 0, 0) x (0, 1, 0) in component "04_Torretta_parte_fissa_azimut"
sketch "Schizzo12 (4)" plane through (36, 0, 0) normal (1, 0, 0) x (0, 0, -1) in component "04_Torretta_parte_fissa_azimut"
  line L0 (-63.9, -8.15) -> (-68.4, -8.15)
  line L1 (-68.4, -8.15) -> (-68.4, -3.15)
  line L2 (-68.4, -3.15) -> (-63.9, -3.15)
  line L3 (-63.9, -3.15) -> (-63.9, -8.15)
extrude "Diramazione_cavo_5x4_5_SG90_Destra" cut sketch "Schizzo12 (4)" along normal blind 4 bodies 7 in component "04_Torretta_parte_fissa_azimut"
ref_plane "Piano di lavoro8" through (0, 0, 65.9) normal (0, 0, 1) x (1, 0, 0) in component "04_Torretta_parte_fissa_azimut"
sketch "Schizzo13 (3)" plane through (0, 0, 65.9) normal (0, 0, 1) x (1, 0, 0) in component "04_Torretta_parte_fissa_azimut"
  line L0 (-63.5, -24.8) -> (-40, -24.8)
  line L1 (-40, -24.8) -> (-40, 13.5)
  line L2 (-40, 13.5) -> (-63.5, 13.5)
  line L3 (-63.5, 13.5) -> (-63.5, -24.8)
extrude "Estrusione_Slitta_SG90_Sinistra_ripiano_Inferiore" add sketch "Schizzo13 (3)" along normal blind 2.5 bodies 7 in component "04_Torretta_parte_fissa_azimut"
ref_plane "Piano di lavoro9" through (0, 0, 81.6) normal (0, 0, 1) x (1, 0, 0) in component "04_Torretta_parte_fissa_azimut"
sketch "Schizzo14 (3)" plane through (0, 0, 81.6) normal (0, 0, 1) x (1, 0, 0) in component "04_Torretta_parte_fissa_azimut"
  line L0 (-63.5, -24.8) -> (-40, -24.8)
  line L1 (-40, -24.8) -> (-40, 13.5)
  line L2 (-40, 13.5) -> (-63.5, 13.5)
  line L3 (-63.5, 13.5) -> (-63.5, -24.8)
extrude "Estrusione_Slitta_SG90_Sinistra_ripiano_Superiore" add sketch "Schizzo14 (3)" along normal blind 2.5 bodies 7 in component "04_Torretta_parte_fissa_azimut"
ref_plane "Piano di lavoro10" through (0, 0, 65.9) normal (0, 0, 1) x (1, 0, 0) in component "04_Torretta_parte_fissa_azimut"
sketch "Schizzo15 (3)" plane through (0, 0, 65.9) normal (0, 0, 1) x (1, 0, 0) in component "04_Torretta_parte_fissa_azimut"
  line L0 (-63.5, -8.15) -> (-61.5, -8.15)
  line L1 (-61.5, -8.15) -> (-61.5, -3.15)
  line L2 (-61.5, -3.15) -> (-63.5, -3.15)
  line L3 (-63.5, -3.15) -> (-63.5, -8.15)
extrude "Uscita_cavo_5x2_SG90_Sinistra" cut sketch "Schizzo15 (3)" along normal blind 2.5 bodies 7 in component "04_Torretta_parte_fissa_azimut"
ref_plane "Piano di lavoro11" through (-63.5, 0, 0) normal (1, 0, 0) x (0, 1, 0) in component "04_Torretta_parte_fissa_azimut"
sketch "Schizzo16 (3)" plane through (-63.5, 0, 0) normal (1, 0, 0) x (0, 0, -1) in component "04_Torretta_parte_fissa_azimut"
  line L0 (-68.4, -24.8) -> (-81.6, -24.8)
  line L1 (-81.6, -24.8) -> (-81.6, -22.3)
  line L2 (-81.6, -22.3) -> (-68.4, -22.3)
  line L3 (-68.4, -22.3) -> (-68.4, -24.8)
extrude "Estrusione_Slitta_SG90_Sinistra_guida_01" add sketch "Schizzo16 (3)" along normal blind 23.5 bodies 7 in component "04_Torretta_parte_fissa_azimut"
ref_plane "Piano di lavoro12" through (-63.5, 0, 0) normal (1, 0, 0) x (0, 1, 0) in component "04_Torretta_parte_fissa_azimut"
sketch "Schizzo17 (3)" plane through (-63.5, 0, 0) normal (1, 0, 0) x (0, 0, -1) in component "04_Torretta_parte_fissa_azimut"
  line L0 (-68.4, 11) -> (-81.6, 11)
  line L1 (-81.6, 11) -> (-81.6, 13.5)
  line L2 (-81.6, 13.5) -> (-68.4, 13.5)
  line L3 (-68.4, 13.5) -> (-68.4, 11)
extrude "Estrusione_Slitta_SG90_Sinistra_guida_02" add sketch "Schizzo17 (3)" along normal blind 23.5 bodies 7 in component "04_Torretta_parte_fissa_azimut"
ref_plane "Piano di lavoro13" through (-63.5, 0, 0) normal (1, 0, 0) x (0, 1, 0) in component "04_Torretta_parte_fissa_azimut"
sketch "Schizzo18 (2)" plane through (-63.5, 0, 0) normal (1, 0, 0) x (0, 0, -1) in component "04_Torretta_parte_fissa_azimut"
  circle A0 centre (-75, -23.55) radius 1.1
extrude "Preforo_M2_5_slitta_Sinistra_01" cut sketch "Schizzo18 (2)" along normal blind 23.5 bodies 7 in component "04_Torretta_parte_fissa_azimut"
ref_plane "Piano di lavoro14" through (-63.5, 0, 0) normal (1, 0, 0) x (0, 1, 0) in component "04_Torretta_parte_fissa_azimut"
sketch "Schizzo19 (2)" plane through (-63.5, 0, 0) normal (1, 0, 0) x (0, 0, -1) in component "04_Torretta_parte_fissa_azimut"
  circle A0 centre (-75, 12.25) radius 1.1
extrude "Preforo_M2_5_slitta_Sinistra_02" cut sketch "Schizzo19 (2)" along normal blind 23.5 bodies 7 in component "04_Torretta_parte_fissa_azimut"
ref_plane "Piano di lavoro15" through (0, 0, 65.9) normal (0, 0, 1) x (1, 0, 0) in component "04_Torretta_parte_fissa_azimut"
sketch "Schizzo20 (2)" plane through (0, 0, 65.9) normal (0, 0, 1) x (1, 0, 0) in component "04_Torretta_parte_fissa_azimut"
  line L0 (40, -24.8) -> (63.5, -24.8)
  line L1 (63.5, -24.8) -> (63.5, 13.5)
  line L2 (63.5, 13.5) -> (40, 13.5)
  line L3 (40, 13.5) -> (40, -24.8)
extrude "Estrusione_Slitta_SG90_Destra_ripiano_Inferiore" add sketch "Schizzo20 (2)" along normal blind 2.5 bodies 7 in component "04_Torretta_parte_fissa_azimut"
ref_plane "Piano di lavoro16" through (0, 0, 81.6) normal (0, 0, 1) x (1, 0, 0) in component "04_Torretta_parte_fissa_azimut"
sketch "Schizzo21 (2)" plane through (0, 0, 81.6) normal (0, 0, 1) x (1, 0, 0) in component "04_Torretta_parte_fissa_azimut"
  line L0 (40, -24.8) -> (63.5, -24.8)
  line L1 (63.5, -24.8) -> (63.5, 13.5)
  line L2 (63.5, 13.5) -> (40, 13.5)
  line L3 (40, 13.5) -> (40, -24.8)
extrude "Estrusione_Slitta_SG90_Destra_ripiano_Superiore" add sketch "Schizzo21 (2)" along normal blind 2.5 bodies 7 in component "04_Torretta_parte_fissa_azimut"
ref_plane "Piano di lavoro17" through (0, 0, 65.9) normal (0, 0, 1) x (1, 0, 0) in component "04_Torretta_parte_fissa_azimut"
sketch "Schizzo22" plane through (0, 0, 65.9) normal (0, 0, 1) x (1, 0, 0) in component "04_Torretta_parte_fissa_azimut"
  line L0 (61.5, -8.15) -> (63.5, -8.15)
  line L1 (63.5, -8.15) -> (63.5, -3.15)
  line L2 (63.5, -3.15) -> (61.5, -3.15)
  line L3 (61.5, -3.15) -> (61.5, -8.15)
extrude "Uscita_cavo_5x2_SG90_Destra" cut sketch "Schizzo22" along normal blind 2.5 bodies 7 in component "04_Torretta_parte_fissa_azimut"
ref_plane "Piano di lavoro18" through (40, 0, 0) normal (1, 0, 0) x (0, 1, 0) in component "04_Torretta_parte_fissa_azimut"
sketch "Schizzo23" plane through (40, 0, 0) normal (1, 0, 0) x (0, 0, -1) in component "04_Torretta_parte_fissa_azimut"
  line L0 (-68.4, -24.8) -> (-81.6, -24.8)
  line L1 (-81.6, -24.8) -> (-81.6, -22.3)
  line L2 (-81.6, -22.3) -> (-68.4, -22.3)
  line L3 (-68.4, -22.3) -> (-68.4, -24.8)
extrude "Estrusione_Slitta_SG90_Destra_guida_01" add sketch "Schizzo23" along normal blind 23.5 bodies 7 in component "04_Torretta_parte_fissa_azimut"
ref_plane "Piano di lavoro19" through (40, 0, 0) normal (1, 0, 0) x (0, 1, 0) in component "04_Torretta_parte_fissa_azimut"
sketch "Schizzo24" plane through (40, 0, 0) normal (1, 0, 0) x (0, 0, -1) in component "04_Torretta_parte_fissa_azimut"
  line L0 (-68.4, 11) -> (-81.6, 11)
  line L1 (-81.6, 11) -> (-81.6, 13.5)
  line L2 (-81.6, 13.5) -> (-68.4, 13.5)
  line L3 (-68.4, 13.5) -> (-68.4, 11)
extrude "Estrusione_Slitta_SG90_Destra_guida_02" add sketch "Schizzo24" along normal blind 23.5 bodies 7 in component "04_Torretta_parte_fissa_azimut"
ref_plane "Piano di lavoro20" through (40, 0, 0) normal (1, 0, 0) x (0, 1, 0) in component "04_Torretta_parte_fissa_azimut"
sketch "Schizzo25" plane through (40, 0, 0) normal (1, 0, 0) x (0, 0, -1) in component "04_Torretta_parte_fissa_azimut"
  circle A0 centre (-75, -23.55) radius 1.1
extrude "Preforo_M2_5_slitta_Destra_01" cut sketch "Schizzo25" along normal blind 23.5 bodies 7 in component "04_Torretta_parte_fissa_azimut"
ref_plane "Piano di lavoro21" through (40, 0, 0) normal (1, 0, 0) x (0, 1, 0) in component "04_Torretta_parte_fissa_azimut"
sketch "Schizzo26" plane through (40, 0, 0) normal (1, 0, 0) x (0, 0, -1) in component "04_Torretta_parte_fissa_azimut"
  circle A0 centre (-75, 12.25) radius 1.1
extrude "Preforo_M2_5_slitta_Destra_02" cut sketch "Schizzo26" along normal blind 23.5 bodies 7 in component "04_Torretta_parte_fissa_azimut"
ref_plane "Piano di lavoro1" through (-63, 0, 0) normal (1, 0, 0) x (0, 1, 0) in component "05_Servo_TowerPro_SG90_Sinistro_riferimento"
sketch "Schizzo1 (9)" plane through (-63, 0, 0) normal (1, 0, 0) x (0, 0, -1) in component "05_Servo_TowerPro_SG90_Sinistro_riferimento"
  line L0 (-68.9, -17) -> (-81.1, -17)
  line L1 (-81.1, -17) -> (-81.1, 5.7)
  line L2 (-81.1, 5.7) -> (-68.9, 5.7)
  line L3 (-68.9, 5.7) -> (-68.9, -17)
extrude "Estrusione_Corpo_SG90_Sinistro" add sketch "Schizzo1 (9)" along normal blind 27 separate body makes body 8 in component "05_Servo_TowerPro_SG90_Sinistro_riferimento"
ref_plane "Piano di lavoro2" through (-36, 0, 0) normal (1, 0, 0) x (0, 1, 0) in component "05_Servo_TowerPro_SG90_Sinistro_riferimento"
sketch "Schizzo2 (8)" plane through (-36, 0, 0) normal (1, 0, 0) x (0, 0, -1) in component "05_Servo_TowerPro_SG90_Sinistro_riferimento"
  circle A0 centre (-75, 0) radius 3
extrude "Estrusione_Albero_uscita_SG90_Sinistro" add sketch "Schizzo2 (8)" along normal blind 3.3 bodies 8 in component "05_Servo_TowerPro_SG90_Sinistro_riferimento"
ref_plane "Piano di lavoro1" through (36, 0, 0) normal (1, 0, 0) x (0, 1, 0) in component "06_Servo_TowerPro_SG90_Destro_riferimento"
sketch "Schizzo1 (10)" plane through (36, 0, 0) normal (1, 0, 0) x (0, 0, -1) in component "06_Servo_TowerPro_SG90_Destro_riferimento"
  line L0 (-68.9, -17) -> (-81.1, -17)
  line L1 (-81.1, -17) -> (-81.1, 5.7)
  line L2 (-81.1, 5.7) -> (-68.9, 5.7)
  line L3 (-68.9, 5.7) -> (-68.9, -17)
extrude "Estrusione_Corpo_SG90_Destro" add sketch "Schizzo1 (10)" along normal blind 27 separate body makes body 9 in component "06_Servo_TowerPro_SG90_Destro_riferimento"
ref_plane "Piano di lavoro2" through (32.7, 0, 0) normal (1, 0, 0) x (0, 1, 0) in component "06_Servo_TowerPro_SG90_Destro_riferimento"
sketch "Schizzo2 (9)" plane through (32.7, 0, 0) normal (1, 0, 0) x (0, 0, -1) in component "06_Servo_TowerPro_SG90_Destro_riferimento"
  circle A0 centre (-75, 0) radius 3
extrude "Estrusione_Albero_uscita_SG90_Destro" add sketch "Schizzo2 (9)" along normal blind 3.3 bodies 9 in component "06_Servo_TowerPro_SG90_Destro_riferimento"
ref_plane "Piano di lavoro1" through (-66.5, 0, 0) normal (1, 0, 0) x (0, 1, 0) in component "07_Barrette_removibili_M2_5_SG90_Sinistra"
sketch "Schizzo1 (11)" plane through (-66.5, 0, 0) normal (1, 0, 0) x (0, 0, -1) in component "07_Barrette_removibili_M2_5_SG90_Sinistra"
  line L0 (-68.4, -24.8) -> (-81.6, -24.8)
  line L1 (-81.6, -24.8) -> (-81.6, -14)
  line L2 (-81.6, -14) -> (-68.4, -14)
  line L3 (-68.4, -14) -> (-68.4, -24.8)
extrude "Estrusione_Barretta_Sinistra_01" add sketch "Schizzo1 (11)" along normal blind 3 separate body makes body 10 in component "07_Barrette_removibili_M2_5_SG90_Sinistra"
ref_plane "Piano di lavoro2" through (-66.5, 0, 0) normal (1, 0, 0) x (0, 1, 0) in component "07_Barrette_removibili_M2_5_SG90_Sinistra"
sketch "Schizzo2 (10)" plane through (-66.5, 0, 0) normal (1, 0, 0) x (0, 0, -1) in component "07_Barrette_removibili_M2_5_SG90_Sinistra"
  circle A0 centre (-75, -23.55) radius 1.35
extrude "Foro_M2_5_barretta_Sinistra_01" cut sketch "Schizzo2 (10)" along normal blind 3 bodies 10 in component "07_Barrette_removibili_M2_5_SG90_Sinistra"
ref_plane "Piano di lavoro3" through (-66.5, 0, 0) normal (1, 0, 0) x (0, 1, 0) in component "07_Barrette_removibili_M2_5_SG90_Sinistra"
sketch "Schizzo3 (8)" plane through (-66.5, 0, 0) normal (1, 0, 0) x (0, 0, -1) in component "07_Barrette_removibili_M2_5_SG90_Sinistra"
  line L0 (-68.4, 2.7) -> (-81.6, 2.7)
  line L1 (-81.6, 2.7) -> (-81.6, 13.5)
  line L2 (-81.6, 13.5) -> (-68.4, 13.5)
  line L3 (-68.4, 13.5) -> (-68.4, 2.7)
extrude "Estrusione_Barretta_Sinistra_02" add sketch "Schizzo3 (8)" along normal blind 3 separate body makes body 11 in component "07_Barrette_removibili_M2_5_SG90_Sinistra"
ref_plane "Piano di lavoro4" through (-66.5, 0, 0) normal (1, 0, 0) x (0, 1, 0) in component "07_Barrette_removibili_M2_5_SG90_Sinistra"
sketch "Schizzo4 (7)" plane through (-66.5, 0, 0) normal (1, 0, 0) x (0, 0, -1) in component "07_Barrette_removibili_M2_5_SG90_Sinistra"
  circle A0 centre (-75, 12.25) radius 1.35
extrude "Foro_M2_5_barretta_Sinistra_02" cut sketch "Schizzo4 (7)" along normal blind 3 bodies 11 in component "07_Barrette_removibili_M2_5_SG90_Sinistra"
ref_plane "Piano di lavoro1" through (63.5, 0, 0) normal (1, 0, 0) x (0, 1, 0) in component "08_Barrette_removibili_M2_5_SG90_Destra"
sketch "Schizzo1 (12)" plane through (63.5, 0, 0) normal (1, 0, 0) x (0, 0, -1) in component "08_Barrette_removibili_M2_5_SG90_Destra"
  line L0 (-68.4, -24.8) -> (-81.6, -24.8)
  line L1 (-81.6, -24.8) -> (-81.6, -14)
  line L2 (-81.6, -14) -> (-68.4, -14)
  line L3 (-68.4, -14) -> (-68.4, -24.8)
extrude "Estrusione_Barretta_Destra_01" add sketch "Schizzo1 (12)" along normal blind 3 separate body makes body 12 in component "08_Barrette_removibili_M2_5_SG90_Destra"
ref_plane "Piano di lavoro2" through (63.5, 0, 0) normal (1, 0, 0) x (0, 1, 0) in component "08_Barrette_removibili_M2_5_SG90_Destra"
sketch "Schizzo2 (11)" plane through (63.5, 0, 0) normal (1, 0, 0) x (0, 0, -1) in component "08_Barrette_removibili_M2_5_SG90_Destra"
  circle A0 centre (-75, -23.55) radius 1.35